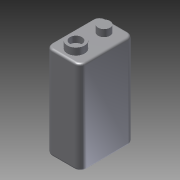
# Autodesk Inventor part: Battery9V
Saved by Autodesk Inventor 2011 SP2 (Build 150309200, 309)
## iProperties
Created: 2015-01-24
Part Number: Battery9V
Document SubType Name: Modeling
Designer: Ernest
Density: 1 g/cm^3
Mass: 18.7097 g
Surface Area: 44.8718 cm^2
Volume: 18.7097 cm^3
Author: Ernest
Autodesk Inventor part; units mm, degrees
ref_plane "YZ Plane" through (0, 0, 0) normal (1, 0, 0) x (0, 1, 0)
ref_plane "XZ Plane" through (0, 0, 0) normal (0, 1, 0) x (-1, 0, 0)
ref_plane "XY Plane" through (0, 0, 0) normal (0, 0, 1) x (1, 0, 0)
sketch "Sketch1" plane through (0, 0, 0) normal (0, 0, 1) x (1, 0, 0)
  line L0 (0, 0) -> (25.7, 0)
  line L1 (25.7, 0) -> (25.7, 44.3)
  line L2 (25.7, 44.3) -> (0, 44.3)
  line L3 (0, 44.3) -> (0, 0)
  dimension "d0" = 25.7
  dimension "d1" = 44.3
  constraints: 8 end point, 2 parallel, 1 horizontal, 1 perpendicular
  measures "d0" distance of L2.end L1.end
  measures "d1" distance of L0.end L1.end
extrude "Extrusion1" add sketch "Sketch1" along normal blind 16.6
sketch "Sketch2" plane through (0, 44.3, 0) normal (0, 1, 0) x (1, 0, 0)
  line L0 (0, 0) -> (0, -16.6) projected
  circle A0 centre (6.15, -8.3) radius 4.15
  circle A1 centre (19.55, -8.3) radius 2.85
  dimension "d4" = 8.3
  dimension "d5" = 5.7
  dimension "d6" = 13.4
  dimension "d7" = 6.15
  constraints: 2 centre point
  measures "d4" diameter of A0
  measures "d5" diameter of A1
  measures "d6" distance of A1.centre A0.centre
  measures "d7" distance from line of L0 A0.centre
extrude "Extrusion2" add sketch "Sketch2" along normal blind 3.3
sketch "Sketch3" plane through (6.15, 47.6, 8.3) normal (0, 1, 0) x (1, 0, 0)
  circle A0 centre (0, 0) radius 4.15 projected
  circle A1 centre (0, 0) radius 2.85
  point P0 (-6.15, 8.3)
  dimension "d10" = 5.7
  constraints: 1 centre point, 1 coincident
  measures "d10" diameter of A1
extrude "Extrusion3" cut sketch "Sketch3" against normal blind 3 contours A1
fillet "Fillet1" radius 3 4 edges at (25.7, 22.15, 16.6) (25.7, 22.15, 0) (0, 22.15, 16.6) (0, 22.15, 0)
fillet "Fillet2" radius 1 16 edges at (12.85, 44.3, 16.6) (24.8213, 44.3, 15.7213) (25.7, 44.3, 8.3) (24.8213, 44.3, 0.8787) (12.85, 44.3, 0) (0.8787, 44.3, 0.8787) (0, 44.3, 8.3) (0.8787, 44.3, 15.7213) (12.85, 0, 16.6) (0.8787, 0, 15.7213) (0, 0, 8.3) (0.8787, 0, 0.8787) (12.85, 0, 0) (24.8213, 0, 0.8787) (25.7, 0, 8.3) (24.8213, 0, 15.7213)
body "Solid1"
